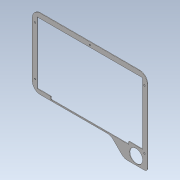
# Autodesk Inventor part: Лицевой лист
Saved by Autodesk Inventor 2021.2 (Build 252289000, 289)
## iProperties
Created: 2022-11-29
Part Number: Лицевой лист
Material: Типовые
Document SubType Name: ЛистМат
Designer: Voodoo
Density: 1 g/cm^3
Sheet Metal Rule: По умолчанию_мм
Appearance: По умолчанию
Mass: 44.314 g
Surface Area: 503.23 cm^2
Volume: 44.314 cm^3
Flat Pattern Width: 31.48 cm
Flat Pattern Length: 43.18 cm
Flat Pattern Area: 1359.31 cm^2
Sheet Metal Width: 314,800 мм
Sheet Metal Length: 431,800 мм
Sheet Metal Area: 135930,640 мм^2
Author: Voodoo
Autodesk Inventor part; units mm, degrees
ref_plane "YZ Plane" through (0, 0, 0) normal (1, 0, 0) x (0, 1, 0)
ref_plane "XZ Plane" through (0, 0, 0) normal (0, 1, 0) x (-1, 0, 0)
ref_plane "XY Plane" through (0, 0, 0) normal (0, 0, 1) x (1, 0, 0)
sketch "Эскиз1" plane through (0, 0, 0) normal (0, 0, 1) x (1, 0, 0)
  line L0 (-186, -134.5) -> (65.5736, -134.5)
  line L1 (218, -134.5) -> (218, 102.5)
  line L2 (186, 134.5) -> (-186, 134.5)
  line L3 (-218, 102.5) -> (-218, -102.5)
  line L4 (-218, -134.5) -> (218, 134.5) construction
  line L5 (218, -134.5) -> (-218, 134.5) construction
  arc A0 (-186, 134.5) -> (-218, 102.5) centre (-186, 102.5) ccw
  arc A1 (218, 102.5) -> (186, 134.5) centre (186, 102.5) ccw
  arc A2 (-218, -102.5) -> (-186, -134.5) centre (-186, -102.5) ccw
  line L6 (218, -134.5) -> (218, -172.5)
  line L7 (206, -184.5) -> (140.4264, -184.5)
  line L8 (119.2132, -175.7132) -> (86.7868, -143.2868)
  arc A3 (206, -184.5) -> (218, -172.5) centre (206, -172.5) ccw
  arc A4 (119.2132, -175.7132) -> (140.4264, -184.5) centre (140.4264, -154.5) ccw
  arc A5 (86.7868, -143.2868) -> (65.5736, -134.5) centre (65.5736, -164.5) ccw
  line L9 (-186, 132.4) -> (186, 132.4)
  arc A6 (215.9, 102.5) -> (186, 132.4) centre (186, 102.5) ccw
  line L10 (215.9, 102.5) -> (215.9, -134.5)
  line L11 (215.9, -134.5) -> (215.9, -172.5)
  arc A7 (206, -182.4) -> (215.9, -172.5) centre (206, -172.5) ccw
  line L12 (206, -182.4) -> (140.4264, -182.4)
  arc A8 (120.6981, -174.2283) -> (140.4264, -182.4) centre (140.4264, -154.5) ccw
  line L13 (120.6981, -174.2283) -> (88.2717, -141.8019)
  arc A9 (88.2717, -141.8019) -> (65.5736, -132.4) centre (65.5736, -164.5) ccw
  line L14 (65.5736, -132.4) -> (-186, -132.4)
  arc A10 (-215.9, -102.5) -> (-186, -132.4) centre (-186, -102.5) ccw
  line L15 (-215.9, -102.5) -> (-215.9, 102.5)
  arc A11 (-186, 132.4) -> (-215.9, 102.5) centre (-186, 102.5) ccw
  point P0 (0, 0)
  point P1 (218, -184.5)
  point P2 (128, -184.5)
  dimension "d2" = 436
  dimension "d3" = 269
  dimension "d4" = 32
  dimension "d5" = 319
  dimension "d6" = 12
  dimension "d7" = 50
  dimension "d8" = 90
  dimension "d9" = 135
  dimension "d10" = 30
  dimension "d11" = 2.1
  constraints: 32 end point, 24 point on circle, 12 centre point, 12 point on line, 12 tangent, 4 parallel, 4 perpendicular, 3 equal radius, 2 midpoint, 1 horizontal, 12 other
  measures "d2" distance of L5.end L4.end
  measures "d3" distance of L4.end L1.start
  measures "d4" radius of A0
  measures "d5" distance between parallel lines of L7 L2
  measures "d6" radius of A3
  measures "d7" distance between parallel lines of L0 L7
  measures "d8" distance from line of L6 point (128, -184.5)
  measures "d9" angle of L0 L8
  measures "d10" radius of A4
  measures "d11" distance between parallel lines of L2 L9
extrude "Пластина1" add sketch "Эскиз1" along normal blind 2 contours L9 A6 L10 L11 A7 L12 A8 L13 A9 L14 A10 L15 A11
sketch "Эскиз2" plane through (0, 0, 0) normal (0, 0, -1) x (-1, 0, 0)
  line L0 (-191.1, 107.6) -> (190.9, 107.6) construction
  line L1 (190.9, 107.6) -> (190.9, -107.4) construction
  line L2 (190.9, -107.4) -> (-191.1, -107.4) construction
  line L3 (-191.1, -107.4) -> (-191.1, 107.6) construction
  line L4 (215.9, -102.5) -> (215.9, 102.5) projected
  line L5 (-65.5736, -132.4) -> (186, -132.4) projected
  line L6 (-197.1, 114.6) -> (196.9, 114.6)
  line L7 (197.9, 113.6) -> (197.9, -117.4)
  line L8 (-147.1, -118.4) -> (-197.1, -118.4)
  line L9 (-198.1, -117.4) -> (-198.1, 113.6)
  line L10 (-146.1, -118.4) -> (145.9, -118.4) construction
  line L11 (145.9, -119.4) -> (145.9, -127.4)
  line L12 (144.9, -128.4) -> (-145.1, -128.4)
  line L13 (-146.1, -127.4) -> (-146.1, -119.4)
  arc A0 (196.9, -118.4) -> (197.9, -117.4) centre (196.9, -117.4) ccw
  arc A1 (197.9, 113.6) -> (196.9, 114.6) centre (196.9, 113.6) ccw
  arc A2 (-197.1, 114.6) -> (-198.1, 113.6) centre (-197.1, 113.6) ccw
  arc A3 (-198.1, -117.4) -> (-197.1, -118.4) centre (-197.1, -117.4) ccw
  arc A4 (-146.1, -127.4) -> (-145.1, -128.4) centre (-145.1, -127.4) ccw
  arc A5 (-146.1, -119.4) -> (-147.1, -118.4) centre (-147.1, -119.4) ccw
  line L14 (146.9, -118.4) -> (196.9, -118.4)
  arc A6 (146.9, -118.4) -> (145.9, -119.4) centre (146.9, -119.4) ccw
  arc A7 (144.9, -128.4) -> (145.9, -127.4) centre (144.9, -127.4) ccw
  point P0 (0, 0)
  point P1 (-198.1, 114.6)
  point P2 (197.9, -118.4)
  point P3 (197.9, 114.6)
  dimension "d13" = 25
  dimension "d14" = 25
  dimension "d15" = 215
  dimension "d16" = 382
  dimension "d24" = 233
  dimension "d25" = 7
  dimension "d26" = 7
  dimension "d27" = 396
  dimension "d28" = 4
  dimension "d29" = 52
  dimension "d30" = 292
  dimension "d31" = 1
  dimension "d32" = 1
  dimension "d33" = 1
  constraints: 26 end point, 17 tangent, 16 point on circle, 11 point on line, 8 centre point, 6 parallel, 5 equal radius, 4 horizontal, 3 perpendicular
  measures "d13" distance between parallel lines of L4 L1
  measures "d14" distance between parallel lines of L5 L2
  measures "d15" distance of L0.end L1.end
  measures "d16" distance of L0.start L0.end
  measures "d24" distance of point (197.9, 114.6) point (197.9, -118.4)
  measures "d25" distance between parallel lines of L6 L0
  measures "d26" distance between parallel lines of L7 L1
  measures "d27" distance of point (-198.1, 114.6) point (197.9, 114.6)
  measures "d28" distance between parallel lines of L12 L5
  measures "d29" distance between parallel lines of L9 L13
  measures "d30" distance between parallel lines of L13 L11
  measures "d31" radius of A0
  measures "d32" radius of A6
  measures "d33" radius of A7
extrude "Вырез1" cut sketch "Эскиз2" against normal blind 2
sketch "Эскиз3" plane through (0, 0, 0) normal (0, 0, -1) x (-1, 0, 0)
  line L0 (186, 132.4) -> (-186, 132.4) projected
  arc A0 (-186, 132.4) -> (-215.9, 102.5) centre (-186, 102.5) ccw projected
  line L1 (-215.9, 102.5) -> (-215.9, -172.5) projected
  arc A1 (-215.9, -172.5) -> (-206, -182.4) centre (-206, -172.5) ccw projected
  line L2 (-206, -182.4) -> (-140.4264, -182.4) projected
  arc A2 (-140.4264, -182.4) -> (-120.6981, -174.2283) centre (-140.4264, -154.5) ccw projected
  line L3 (-120.6981, -174.2283) -> (-88.2717, -141.8019) projected
  arc A3 (-65.5736, -132.4) -> (-88.2717, -141.8019) centre (-65.5736, -164.5) ccw projected
  line L4 (-65.5736, -132.4) -> (186, -132.4) projected
  arc A4 (186, -132.4) -> (215.9, -102.5) centre (186, -102.5) ccw projected
  line L5 (215.9, -102.5) -> (215.9, 102.5) projected
  arc A5 (215.9, 102.5) -> (186, 132.4) centre (186, 102.5) ccw projected
  circle A6 centre (-173.9, -152.4) radius 25
  point P0 (0, 0)
  dimension "d19" = 50
  dimension "d20" = 30
  dimension "d21" = 42
  constraints: 1 centre point
  measures "d19" diameter of A6
  measures "d20" distance from line of A6.centre L2
  measures "d21" distance from line of A6.centre L1
extrude "Вырез2" cut sketch "Эскиз3" against normal blind 2 contours A6
sketch "Эскиз4" plane through (0, 0, 2) normal (0, 0, 1) x (1, 0, 0)
  circle A0 centre (173.9, -152.4) radius 25 projected
  arc A1 (-196.9, 114.6) -> (-197.9, 113.6) centre (-196.9, 113.6) ccw projected
  line L0 (-196.9, 114.6) -> (197.1, 114.6) projected
  arc A2 (198.1, 113.6) -> (197.1, 114.6) centre (197.1, 113.6) ccw projected
  line L1 (198.1, 113.6) -> (198.1, -117.4) projected
  arc A3 (197.1, -118.4) -> (198.1, -117.4) centre (197.1, -117.4) ccw projected
  line L2 (197.1, -118.4) -> (147.1, -118.4) projected
  arc A4 (147.1, -118.4) -> (146.1, -119.4) centre (147.1, -119.4) ccw projected
  line L3 (146.1, -119.4) -> (146.1, -127.4) projected
  arc A5 (145.1, -128.4) -> (146.1, -127.4) centre (145.1, -127.4) ccw projected
  line L4 (145.1, -128.4) -> (-144.9, -128.4) projected
  arc A6 (-145.9, -127.4) -> (-144.9, -128.4) centre (-144.9, -127.4) ccw projected
  line L5 (-145.9, -127.4) -> (-145.9, -119.4) projected
  arc A7 (-145.9, -119.4) -> (-146.9, -118.4) centre (-146.9, -119.4) ccw projected
  line L6 (-146.9, -118.4) -> (-196.9, -118.4) projected
  arc A8 (-197.9, -117.4) -> (-196.9, -118.4) centre (-196.9, -117.4) ccw projected
  line L7 (-197.9, -117.4) -> (-197.9, 113.6) projected
  arc A9 (215.9, 102.5) -> (186, 132.4) centre (186, 102.5) ccw projected
  line L8 (-186, 132.4) -> (186, 132.4) projected
  arc A10 (-186, 132.4) -> (-215.9, 102.5) centre (-186, 102.5) ccw projected
  line L9 (-215.9, -102.5) -> (-215.9, 102.5) projected
  arc A11 (-215.9, -102.5) -> (-186, -132.4) centre (-186, -102.5) ccw projected
  line L10 (65.5736, -132.4) -> (-186, -132.4) projected
  arc A12 (88.2717, -141.8019) -> (65.5736, -132.4) centre (65.5736, -164.5) ccw projected
  line L11 (120.6981, -174.2283) -> (88.2717, -141.8019) projected
  arc A13 (120.6981, -174.2283) -> (140.4264, -182.4) centre (140.4264, -154.5) ccw projected
  line L12 (206, -182.4) -> (140.4264, -182.4) projected
  arc A14 (206, -182.4) -> (215.9, -172.5) centre (206, -172.5) ccw projected
  line L13 (215.9, 102.5) -> (215.9, -172.5) projected
  circle A15 centre (-204.9, -91.4) radius 2.1
  circle A16 centre (-204.9, 92.6) radius 2.1
  circle A17 centre (0, 121.6) radius 2.1
  circle A18 centre (205.1, 92.6) radius 2.1
  circle A19 centre (205.1, -128.4) radius 2.1
  line L14 (-202.35, 91.1278) -> (-204.9, 89.6555)
  line L15 (-204.9, 89.6555) -> (-207.45, 91.1278)
  line L16 (-207.45, 91.1278) -> (-207.45, 94.0722)
  line L17 (-207.45, 94.0722) -> (-204.9, 95.5445)
  line L18 (-204.9, 95.5445) -> (-202.35, 94.0722)
  line L19 (-202.35, 94.0722) -> (-202.35, 91.1278)
  line L20 (2.55, 120.1278) -> (0, 118.6555)
  line L21 (0, 118.6555) -> (-2.55, 120.1278)
  line L22 (-2.55, 120.1278) -> (-2.55, 123.0722)
  line L23 (-2.55, 123.0722) -> (0, 124.5445)
  line L24 (0, 124.5445) -> (2.55, 123.0722)
  line L25 (2.55, 123.0722) -> (2.55, 120.1278)
  line L26 (207.65, 91.1278) -> (205.1, 89.6555)
  line L27 (205.1, 89.6555) -> (202.55, 91.1278)
  line L28 (202.55, 91.1278) -> (202.55, 94.0722)
  line L29 (202.55, 94.0722) -> (205.1, 95.5445)
  line L30 (205.1, 95.5445) -> (207.65, 94.0722)
  line L31 (207.65, 94.0722) -> (207.65, 91.1278)
  line L32 (207.65, -129.8722) -> (205.1, -131.3445)
  line L33 (205.1, -131.3445) -> (202.55, -129.8722)
  line L34 (202.55, -129.8722) -> (202.55, -126.9278)
  line L35 (202.55, -126.9278) -> (205.1, -125.4555)
  line L36 (205.1, -125.4555) -> (207.65, -126.9278)
  line L37 (207.65, -126.9278) -> (207.65, -129.8722)
  line L38 (-202.35, -92.8722) -> (-204.9, -94.3445)
  line L39 (-204.9, -94.3445) -> (-207.45, -92.8722)
  line L40 (-207.45, -92.8722) -> (-207.45, -89.9278)
  line L41 (-207.45, -89.9278) -> (-204.9, -88.4555)
  line L42 (-204.9, -88.4555) -> (-202.35, -89.9278)
  line L43 (-202.35, -89.9278) -> (-202.35, -92.8722)
  point P0 (0, 0)
  point P1 (0, 132.4)
  dimension "d34" = 4.2
  dimension "d35" = 4.2
  dimension "d36" = 4.2
  dimension "d37" = 4.2
  dimension "d38" = 4.2
  dimension "d41" = 7
  dimension "d42" = 7
  dimension "d44" = 184
  dimension "d45" = 22
  dimension "d46" = 7
  dimension "d47" = 7
  dimension "d48" = 7
  dimension "d49" = 10
  dimension "d52" = 5.1
  dimension "d53" = 5.1
  dimension "d54" = 5.1
  dimension "d55" = 5.1
  dimension "d56" = 5.1
  constraints: 60 end point, 6 vertical alignment, 5 centre point, 5 coincident, 1 horizontal alignment, 1 midpoint, 65 other
  measures "d34" diameter of A15
  measures "d35" diameter of A16
  measures "d36" diameter of A17
  measures "d37" diameter of A18
  measures "d38" diameter of A19
  measures "d41" distance from line of A16.centre L7
  measures "d42" distance from line of A15.centre L7
  measures "d44" distance of A16.centre A15.centre
  measures "d45" distance from line of A16.centre L0
  measures "d46" distance from line of A17.centre L0
  measures "d47" distance from line of L1 A18.centre
  measures "d48" distance from line of A19.centre L1
  measures "d49" distance from line of A19.centre L2
  measures "d52" distance between parallel lines of L19 L16
  measures "d53" distance between parallel lines of L25 L22
  measures "d54" distance between parallel lines of L28 L31
  measures "d55" distance between parallel lines of L37 L34
  measures "d56" distance between parallel lines of L43 L40
extrude "Вырез3" cut sketch "Эскиз4" against normal blind 2 contours L14 L15 L16 L17 L18 L19 | L20 L21 L22 L23 L24 L25 | L26 L27 L28 L29 L30 L31 | L32 L33 L34 L35 L36 L37 | L38 L39 L40 L41 L42 L43
equation "\"d14\" = d13"
equation "\"d17\" = Толщина"
equation "\"d22\" = Толщина"
equation "\"d34\" = d35"
equation "\"d36\" = d35"
equation "\"d37\" = d36"
equation "\"d38\" = d37"
equation "\"d42\" = d41"
equation "\"d48\" = d47"
equation "\"d54\" = d53"
equation "\"d55\" = d54"
equation "\"d56\" = d52"
equation "\"d50\" = Толщина"
equation "\"d12\" = Толщина"
equation "\"Радиус_гибки\" = Толщина"
equation "\"Ширина_просечки\" = Толщина"
equation "\"Глубина_просечки\" = 0.5 * Толщина"
equation "\"Размер_просечки\" = 4 * Толщина"
equation "\"Мин_остаток\" = 2 * Толщина"
equation "\"Радиус_перехода\" = Радиус_гибки"
equation "\"Радиус_Якоби\" = Радиус_гибки"
equation "\"Размер_зазора\" = Толщина"
equation "\"Толщина\" = 2"
